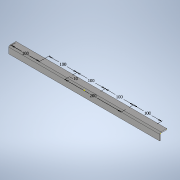
# Autodesk Inventor part: SP33V1 Tope Base
Saved by Autodesk Inventor 2021.2 (Build 252289000, 289)
## iProperties
Created: 2026-08-18
Part Number: SP33V1 Tope Base
Material: Generic
Document SubType Name: Sheet Metal
Designer: nelso
Density: 1 g/cm^3
Sheet Metal Rule: Default_mm
Appearance: Default
Author: nelso
Autodesk Inventor part; units mm, degrees
ref_plane "YZ Plane" through (0, 0, 0) normal (1, 0, 0) x (0, 1, 0)
ref_plane "XZ Plane" through (0, 0, 0) normal (0, 1, 0) x (-1, 0, 0)
ref_plane "XY Plane" through (0, 0, 0) normal (0, 0, 1) x (1, 0, 0)
sketch "Sketch1" plane through (0, 0, 0) normal (0, 1, 0) x (-1, 0, 0)
  line L0 (-267.5, 12.7) -> (267.5, 12.7)
  line L1 (267.5, 12.7) -> (267.5, -12.7)
  line L2 (267.5, -12.7) -> (-267.5, -12.7)
  line L3 (-267.5, -12.7) -> (-267.5, 12.7)
  line L4 (-267.5, 12.7) -> (267.5, -12.7) construction
  line L5 (267.5, 12.7) -> (-267.5, -12.7) construction
  point P0 (0, 0)
  dimension "d0" = 535
  dimension "d1" = 25.4
  measures "d0" distance of L1.end L2.end
  measures "d1" distance of L0.end L1.end
extrude "Plate1" add sketch "Sketch1" along normal blind 3.2
sketch "Sketch2" plane through (267.5, 0, 9.5) normal (0, 0, 1) x (1, 0, 0)
  line L0 (-535, 0) -> (0, 0)
  line L1 (0, 0) -> (0, 25.4)
  line L2 (0, 25.4) -> (-535, 25.4)
  line L3 (-535, 25.4) -> (-535, 0)
  constraints: 6 end point, 1 horizontal, 1 perpendicular, 1 vertical
edge flange "Flange1" height 25.4 angle 90 thickness 3.2 bend radius 1.516 thickness toward (0, 0, 1) relief straight relief width 3.2 relief depth 1.6 edges at (0, 3.2, 12.7) wall of the first edge with corners at (-267.5, 0, 9.5) (267.5, 0, 9.5) (267.5, 25.4, 9.5) (-267.5, 25.4, 9.5)
bend "Bend1"
corner "Corner1"
equation "\"d2\" = Thickness"
equation "\"d3\" = BendReliefWidth"
equation "\"d4\" = BendReliefDepth"
equation "\"d5\" = MinimumRemnant"
equation "\"d6\" = TransitionRadius"
equation "\"d9\" = BendRadius"
equation "\"d10\" = CornerReliefSize"
equation "\"d11\" = GapSize"
equation "\"d12\" = JacobiRadiusSize"
equation "\"BendReliefWidth\" = Thickness"
equation "\"BendReliefDepth\" = 0.5 * Thickness"
equation "\"CornerReliefSize\" = 4 * Thickness"
equation "\"MinimumRemnant\" = 2 * Thickness"
equation "\"TransitionRadius\" = BendRadius"
equation "\"JacobiRadiusSize\" = BendRadius"
equation "\"GapSize\" = Thickness"
equation "\"Thickness\" = 3.2"
equation "\"BendRadius\" = 1.516"
body "Solid1"
